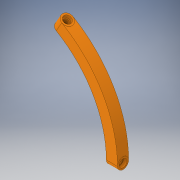
# Autodesk Inventor part: Link2
Saved by Autodesk Inventor 2019 (Build 230136000, 136)
## iProperties
Created: 2022-07-14
Part Number: Link2
Material: Generic
Document SubType Name: Modeling
Designer: zreik
Density: 1 g/cm^3
Appearance: Orange
Author: zreik
Autodesk Inventor part; units mm, degrees
ref_plane "YZ Plane" through (0, 0, 0) normal (1, 0, 0) x (0, 1, 0)
ref_plane "XZ Plane" through (0, 0, 0) normal (0, 1, 0) x (-1, 0, 0)
ref_plane "XY Plane" through (0, 0, 0) normal (0, 0, 1) x (1, 0, 0)
sketch "Sketch1" plane through (0, 0, 0) normal (0, 0, 1) x (1, 0, 0)
  arc A0 (100, 0) -> (50, 86.60254) centre (0, 0) ccw
  line L0 (100, 0) -> (0, 0)
  line L1 (0, 0) -> (50, 86.60254)
  arc A1 (90, 0) -> (45, 77.942286) centre (0, 0) ccw
  dimension "d0" = 60
  dimension "d1" = 100
  dimension "d2" = 10
  constraints: 4 end point, 4 point on circle, 2 centre point, 2 coincident, 2 point on line, 1 horizontal
  measures "d0" angle of L1 L0
  measures "d1" radius of A0
  measures "d2" radial gap between concentric circles of A1 A0
extrude "Extrusion1" add sketch "Sketch1" along normal blind 10 contours L0 A1 L1 A0
ref_plane "Work Plane1" through (50, 86.60254, 0) normal (0.5, 0.8660254, 0) x (-0.8660254, 0.5, 0)
sketch "Sketch2" plane through (50, 86.60254, 0) normal (0.5, 0.8660254, 0) x (-0.8660254, 0.5, 0)
  circle A0 centre (0, 5) radius 5
  line L0 (0, 0) -> (0, 10)
  line L1 (-77.942286, 10) -> (0, 10)
  dimension "d5" = 10
  dimension "d6" = 0
  dimension "d7" = 5
  constraints: 1 centre point
  measures "d5" diameter of A0
  measures "d6" distance from line of L0 A0.centre
  measures "d7" distance from line of L1 A0.centre
extrude "Extrusion2" add sketch "Sketch2" against normal blind 10
ref_plane "Work Plane2" through (100, 0, 0) normal (1, 0, 0) x (0, 1, 0)
sketch "Sketch3" plane through (100, 0, 0) normal (1, 0, 0) x (0, 1, 0)
  circle A0 centre (0, 5) radius 5
  line L0 (0, 0) -> (0, 10)
  line L1 (77.942286, 10) -> (77.942286, 10)
  point P0 (0, 0)
  point P1 (77.942286, 10)
  dimension "d10" = 10
  dimension "d11" = 0
  dimension "d12" = 5
  constraints: 1 centre point, 1 coincident
  measures "d10" diameter of A0
  measures "d11" distance from line of L0 A0.centre
extrude "Extrusion3" add sketch "Sketch3" against normal blind 10
sketch "Sketch4" plane through (45, 77.942286, 0) normal (-0.5, -0.8660254, 0) x (0.8660254, -0.5, 0)
  circle A0 centre (0, 5) radius 2.5
  circle A1 centre (0, 5) radius 5 projected
  point P0 (0, 0)
  point P1 (0, 10)
  dimension "d15" = 5
  constraints: 1 centre point, 1 concentric
  measures "d15" diameter of A0
extrude "Extrusion4" cut sketch "Sketch4" along normal through all both and the other way through all contours A0
sketch "Sketch5" plane through (90, 0, 0) normal (-1, 0, 0) x (0, 0, 1)
  circle A0 centre (5, 0) radius 2.5
  arc A1 (0, 0) -> (10, 0) centre (5, 0) ccw projected
  dimension "d18" = 5
  constraints: 1 centre point, 1 concentric
  measures "d18" diameter of A0
extrude "Extrusion5" cut sketch "Sketch5" along normal through all both and the other way through all
sketch "Sketch6" plane through (50, 86.60254, 0) normal (0.5, 0.8660254, 0) x (0.8660254, -0.5, 0)
  circle A0 centre (0, -5) radius 3.5
  circle A1 centre (0, -5) radius 2.5
  arc A2 (0, -10) -> (0, 0) centre (0, -5) ccw projected
  dimension "d21" = 5
  dimension "d22" = 7
  constraints: 2 centre point, 1 coincident, 1 concentric
  measures "d21" diameter of A1
  measures "d22" diameter of A0
extrude "Extrusion6" cut sketch "Sketch6" against normal blind 3
sketch "Sketch7" plane through (45, 77.942286, 0) normal (-0.5, -0.8660254, 0) x (0.8660254, -0.5, 0)
  circle A0 centre (0, 5) radius 3.5
  circle A1 centre (0, 5) radius 2.5
  arc A2 (0, 7.5) -> (0, 2.5) centre (0, 5) ccw projected
  point P0 (0, 0)
  dimension "d25" = 5
  dimension "d26" = 7
  constraints: 2 centre point, 1 coincident, 1 concentric
  measures "d25" diameter of A1
  measures "d26" diameter of A0
extrude "Extrusion7" cut sketch "Sketch7" along normal mid plane 6
sketch "Sketch8" plane through (90, 0, 0) normal (-1, 0, 0) x (0, 0, 1)
  circle A0 centre (5, 0) radius 3.5
  circle A1 centre (5, 0) radius 2.5
  arc A2 (2.5, 0) -> (7.5, 0) centre (5, 0) ccw projected
  point P0 (0, 0)
  dimension "d29" = 7
  dimension "d30" = 5
  constraints: 2 centre point, 1 coincident, 1 concentric
  measures "d29" diameter of A0
  measures "d30" diameter of A1
extrude "Extrusion8" cut sketch "Sketch8" along normal mid plane 6
sketch "Sketch9" plane through (100, 0, 0) normal (1, 0, 0) x (0, 0, -1)
  circle A0 centre (-5, 0) radius 3.5
  circle A1 centre (-5, 0) radius 2.5
  circle A2 centre (-5, 0) radius 2.5 projected
  point P0 (0, 0)
  dimension "d33" = 5
  dimension "d34" = 7
  constraints: 2 centre point, 1 coincident, 1 concentric
  measures "d33" diameter of A1
  measures "d34" diameter of A0
extrude "Extrusion9" cut sketch "Sketch9" against normal blind 3
equation "\"d1\" = radius"
equation "\"d2\" = thickness"
equation "\"d3\" = width"
equation "\"d5\" = width"
equation "\"d7\" = 0.5 * d5"
equation "\"d8\" = thickness"
equation "\"d10\" = width"
equation "\"d12\" = 0.5 * d10"
equation "\"d13\" = thickness"
equation "\"thickness\" = thickness_1"
equation "\"width\" = width_1"
equation "\"radius\" = radius_1"
equation "\"thickness_1\" = 10"
equation "\"width_1\" = 10"
equation "\"radius_1\" = 100"
body "Solid1"
